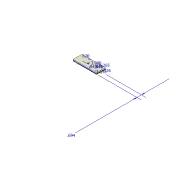
# Autodesk Inventor part: capstone hook mount
Saved by Autodesk Inventor 2020 (Build 240168000, 168)
## iProperties
Created: 2020-02-12
Part Number: capstone hook mount
Material: Generic
Document SubType Name: Modeling
Designer: ball
Density: 1 g/cm^3
Appearance: Default
Author: ball
Autodesk Inventor part; units mm, degrees
ref_plane "XZ Plane" through (0, 0, 0) normal (0, 1, 0) x (-1, 0, 0)
sketch "Sketch1" plane through (0, 0, 0) normal (0, 1, 0) x (-1, 0, 0)
  line L0 (0, 17.637) -> (-76.2, 17.637)
  line L1 (-76.2, 17.637) -> (-76.2, -17.863)
  line L2 (-76.2, -17.863) -> (0, -17.863)
  line L3 (0, -17.863) -> (0, 17.637)
  line L4 (0, 17.637) -> (15.748, 17.637)
  line L5 (15.748, 17.637) -> (15.748, -17.863)
  line L6 (15.748, -17.863) -> (0, -17.863)
  line L7 (0, -17.863) -> (0, 17.637)
  circle A0 centre (-44.068, -12.113) radius 1.7
  circle A1 centre (-68.068, -12.113) radius 1.7
  circle A2 centre (-44.068, 11.887) radius 1.7
  circle A3 centre (-68.068, 11.887) radius 1.7
  point P0 (0, 0)
  dimension "d0" = 76.2
  dimension "d1" = 35.5
  dimension "d2" = 17.637
  dimension "d3" = 15.748
  dimension "d45" = 3.4
  dimension "d46" = 32.132
  dimension "d47" = 5.75
  dimension "d50" = 24
  dimension "d53" = 24
  constraints: 16 end point, 4 centre point, 4 parallel, 3 horizontal, 2 perpendicular, 1 vertical, 6 other
  measures "d0" distance of L2.end L1.end
  measures "d1" distance of L1.end L0.end
  measures "d2" distance from line of L0 point (0, 0)
  measures "d3" distance of L5.end L6.end
  measures "d45" diameter of A0
  measures "d46" distance from line of L1 A0.centre
  measures "d47" distance from line of L2 A0.centre
  measures "d50" distance of A0.centre A1.centre
  measures "d53" distance of A0.centre A2.centre
extrude "Extrusion1" add sketch "Sketch1" along normal blind 4
sketch "Sketch4" plane through (0, 0, 0) normal (0, -1, 0) x (1, 0, 0)
  line L0 (-12.7, 3.175) -> (12.7, 3.175) construction
  line L1 (12.7, 3.175) -> (12.7, -3.175) construction
  line L2 (12.7, -3.175) -> (-12.7, -3.175) construction
  line L3 (-12.7, -3.175) -> (-12.7, 3.175) construction
  line L4 (-6.35, 3.175) -> (-6.35, -3.175) construction
  line L5 (6.35, 3.175) -> (6.35, -3.175) construction
  line L6 (-6.35, 3.683) -> (-13.208, 3.683)
  line L7 (-13.208, 3.683) -> (-13.208, 6.223)
  line L8 (-13.208, 6.223) -> (-6.35, 6.223)
  line L9 (-6.35, 6.223) -> (-6.35, 3.683)
  line L10 (-13.208, 6.223) -> (-15.748, 6.223)
  line L11 (-15.748, 6.223) -> (-15.748, 0)
  line L12 (-15.748, 0) -> (-13.208, 0)
  line L13 (-13.208, 0) -> (-13.208, 6.223)
  line L14 (-12.7, 0) -> (12.7, 0) construction
  line L15 (0, 3.175) -> (0, -3.175) construction
  line L16 (-6.35, -3.683) -> (-13.208, -3.683)
  line L17 (-13.208, -6.223) -> (-6.35, -6.223)
  line L18 (-6.35, -6.223) -> (-6.35, -3.683)
  line L19 (-13.208, -6.223) -> (-15.748, -6.223)
  line L20 (-15.748, -6.223) -> (-15.748, 0)
  line L21 (-13.208, 0) -> (-13.208, -6.223)
  line L22 (6.35, 3.683) -> (13.208, 3.683)
  line L23 (13.208, 3.683) -> (13.208, 6.223)
  line L24 (13.208, 6.223) -> (6.35, 6.223)
  line L25 (6.35, 6.223) -> (6.35, 3.683)
  line L26 (13.208, 6.223) -> (15.748, 6.223)
  line L27 (15.748, 6.223) -> (15.748, 0)
  line L28 (15.748, 0) -> (13.208, 0)
  line L29 (13.208, 0) -> (13.208, 6.223)
  line L30 (6.35, -6.223) -> (6.35, -3.683)
  line L31 (6.35, -3.683) -> (13.208, -3.683)
  line L32 (13.208, -6.223) -> (6.35, -6.223)
  line L33 (13.208, 0) -> (13.208, -6.223)
  line L34 (15.748, -6.223) -> (15.748, 0)
  line L35 (13.208, -6.223) -> (15.748, -6.223)
  point P0 (0, 0)
  dimension "d20" = 25.4
  dimension "d21" = 6.35
  dimension "d22" = 3.175
  dimension "d23" = 12.7
  dimension "d24" = 6.35
  dimension "d25" = 6.35
  dimension "d26" = 6.858
  dimension "d27" = 2.54
  dimension "d28" = 0.508
  dimension "d29" = 2.54
  dimension "d30" = 6.223
  constraints: 72 end point, 17 symmetric about line, 6 parallel, 4 midpoint, 4 perpendicular, 3 horizontal, 2 point on line, 1 collinear
  measures "d20" distance of L1.end L2.end
  measures "d21" distance of L0.end L1.end
  measures "d22" distance from line of L0 point (0, 0)
  measures "d23" distance from line of L3 point (0, 0)
  measures "d24" distance between parallel lines of L4 L3
  measures "d25" distance between parallel lines of L1 L5
  measures "d26" distance of L7.end L8.end
  measures "d27" distance of L6.end L7.end
  measures "d28" distance between parallel lines of L6 L0
  measures "d29" distance of L12.end L11.end
  measures "d30" distance between parallel lines of L12 L10
extrude "Extrusion5" add sketch "Sketch4" along normal blind 6.35
sketch "Sketch6" plane through (0, 0, 0) normal (0, -1, 0) x (1, 0, 0)
  circle A0 centre (27.432, 0) radius 9.525
  line L0 (0, 24.737) -> (0, -24.963) projected
  point P0 (0, 0)
  dimension "d35" = 19.05
  dimension "d36" = 27.432
  constraints: 1 centre point
  measures "d35" diameter of A0
  measures "d36" distance from line of A0.centre L0
extrude "Extrusion7" add sketch "Sketch6" along normal blind 3
sketch "Sketch7" plane through (27.432, -3, 0) normal (0, -1, 0) x (1, 0, 0)
  circle A0 centre (0, 0) radius 1.7
  point P0 (-27.432, 0)
  dimension "d39" = 3.4
  constraints: 1 centre point
  measures "d39" diameter of A0
extrude "Extrusion8" cut sketch "Sketch7" against normal through all
sketch "Sketch8" plane through (0, 0, 0) normal (0, -1, 0) x (1, 0, 0)
  circle A0 centre (27.432, 0) radius 1.7 construction
  line L0 (27.432, 0) -> (15.875, -6.35) construction
  line L1 (27.432, 0) -> (15.875, 0) construction
  line L2 (6.35, -6.223) -> (6.35, -3.683) construction
  line L3 (27.432, 0) -> (6.35, -6.223) construction
  line L4 (27.432, 0) -> (6.35, 3.6065) construction
  point P0 (0, 0)
  constraints: 8 end point
sketch "Sketch9" plane through (0, 4, 0) normal (0, 1, 0) x (1, 0, 0)
  circle A0 centre (27.432, 0) radius 1.7 construction
  circle A1 centre (27.432, 0) radius 3.25 construction
  line L0 (27.432, 3.25) -> (30.2466, 1.625)
  line L1 (30.2466, 1.625) -> (30.2466, -1.625)
  line L2 (30.2466, -1.625) -> (27.432, -3.25)
  line L3 (27.432, -3.25) -> (24.6174, -1.625)
  line L4 (24.6174, -1.625) -> (24.6174, 1.625)
  line L5 (24.6174, 1.625) -> (27.432, 3.25)
  point P0 (0, 0)
  dimension "d42" = 6.5
  constraints: 12 end point, 2 coincident, 1 vertical alignment, 15 other
extrude "Extrusion9" cut sketch "Sketch9" against normal blind 2.5
sketch "Sketch10" plane through (0, 0, 0) normal (0, -1, 0) x (1, 0, 0)
  line L0 (-13.208, 3.683) -> (-13.208, -3.683) projected
  line L1 (13.208, 3.683) -> (6.35, 3.683) projected
  line L2 (-13.208, -3.683) -> (13.208, -3.683)
  line L3 (13.208, -3.683) -> (13.208, 3.683)
  line L4 (13.208, 3.683) -> (-13.208, 3.683)
  line L5 (-13.208, 3.683) -> (-13.208, -3.683)
  point P0 (0, 0)
  constraints: 8 end point, 2 parallel, 1 horizontal, 1 perpendicular
extrude "Extrusion10" add sketch "Sketch10" along normal blind 0.5
equation "\"d22\" = 0.5 * d21"
equation "\"d23\" = 0.5 * d20"
body "Solid1"
